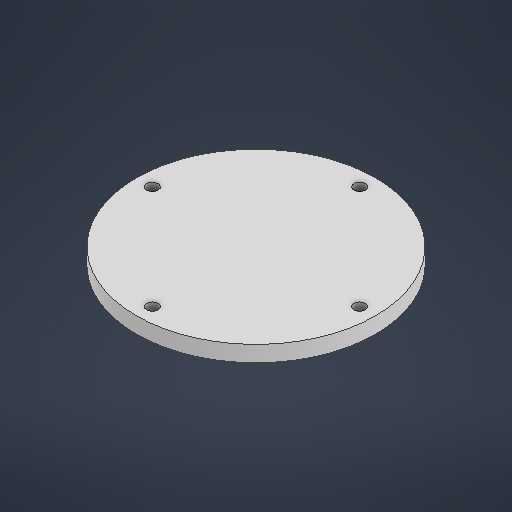
# Autodesk Inventor part: podstava
Saved by Autodesk Inventor 2026 (Build 300175000, 175)
## iProperties
Created: 2025-04-11
Part Number: podstava
Material: Generic
Document SubType Name: Modeling
Designer: vitgr
Density: 1 g/cm^3
Appearance: Default
Author: vitgr
Autodesk Inventor part; units mm, degrees
ref_plane "YZ Plane" through (0, 0, 0) normal (1, 0, 0) x (0, 1, 0)
ref_plane "XZ Plane" through (0, 0, 0) normal (0, 1, 0) x (-1, 0, 0)
ref_plane "XY Plane" through (0, 0, 0) normal (0, 0, 1) x (1, 0, 0)
sketch "Sketch1" plane through (0, 0, 0) normal (0, 1, 0) x (-1, 0, 0)
  circle A0 centre (0, 0) radius 37.5
  dimension "d0" = 75
  constraints: 1 centre point, 1 coincident
  measures "d0" diameter of A0
extrude "Extrusion1" add sketch "Sketch1" along normal blind 5
sketch "Sketch3" plane through (0, 5, 0) normal (0, 1, 0) x (1, 0, 0)
  circle A0 centre (0, 0) radius 37.5 projected
  line L0 (0, 32.5) -> (0, 37.5)
  line L1 (-32.5, 0) -> (-37.5, 0)
  line L2 (0, -32.5) -> (0, -37.5)
  line L3 (32.5, 0) -> (37.5, 0)
  dimension "d6" = 360
  dimension "d10" = 360
  dimension "d12" = 5
  constraints: 8 end point, 1 vertical, 1 vertical alignment, 19 other
  measures "d12" distance of L0.start L0.end
hole "Hole2" at (0, 5, -32.5) at (-32.5, 5, 0) at (0, 5, 32.5) at (32.5, 5, 0) direction (0, -1, 0) diameter 3.6 end through all
body "Solid1"
